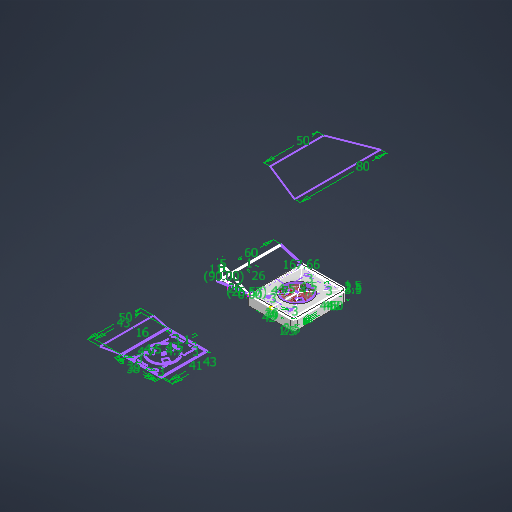
# Autodesk Inventor part: Part1
Saved by Autodesk Inventor 2026 (Build 300175000, 175)
## iProperties
Created: 2025-04-13
Part Number: Part1
Material: Generic
Document SubType Name: Modeling
Designer: ct_vi
Density: 1 g/cm^3
Appearance: Default
Author: ct_vi
Autodesk Inventor part; units mm, degrees
ref_plane "YZ Plane" through (0, 0, 0) normal (1, 0, 0) x (0, 1, 0)
ref_plane "XZ Plane" through (0, 0, 0) normal (0, 1, 0) x (-1, 0, 0)
ref_plane "XY Plane" through (0, 0, 0) normal (0, 0, 1) x (1, 0, 0)
sketch "Sketch1" plane through (0, 0, 0) normal (0, 1, 0) x (-1, 0, 0)
  circle A0 centre (0, 1.5) radius 11.5
  circle A1 centre (0, 1.5) radius 12.5
  line L0 (19.0144, -21.3297) -> (-18.8688, -21.3297) construction
  line L1 (-18.8688, -21.3297) -> (-18.8688, 21.6448) construction
  line L2 (-18.8688, 21.6448) -> (19.0144, 21.6448) construction
  line L3 (19.0144, 21.6448) -> (19.0144, -21.3297) construction
  line L4 (-2.25, -4) -> (-2.25, -8.7)
  line L5 (-2.25, -8.7) -> (2.25, -8.7)
  line L6 (2.25, -8.7) -> (2.25, -4)
  line L7 (2.25, -4) -> (-2.25, -4)
  line L8 (5.9381, 2.2148) -> (9.8353, 4.4648)
  line L9 (9.8353, 4.4648) -> (7.4853, 8.5352)
  line L10 (7.4853, 8.5352) -> (3.5881, 6.2852)
  line L11 (5.9381, 2.2148) -> (3.5881, 6.2852)
  line L12 (-3.5881, 6.2852) -> (-7.4853, 8.5352)
  line L13 (-7.4853, 8.5352) -> (-9.8353, 4.4648)
  line L14 (-9.8353, 4.4648) -> (-5.9381, 2.2148)
  line L15 (-3.5881, 6.2852) -> (-5.9381, 2.2148)
  circle A2 centre (10.199, -17.6855) radius 1.5
  circle A3 centre (-10.301, 18.0645) radius 1.5
  circle A4 centre (10.199, 18.0645) radius 1.5
  circle A5 centre (-10.301, -17.6855) radius 1.5
  line L16 (114.7256, -138.5925) -> (76.7812, -153.4955)
  line L17 (76.7812, -153.4955) -> (76.858, -73.4955)
  line L18 (76.858, -73.4955) -> (114.7256, -88.5925)
  line L19 (114.7256, -88.5925) -> (114.7256, -138.5925)
  line L20 (10.199, -17.6855) -> (-10.301, -17.6855)
  line L21 (-10.301, -17.6855) -> (-10.301, 18.0645)
  line L22 (-10.301, 18.0645) -> (10.199, 18.0645)
  line L23 (10.199, 18.0645) -> (10.199, -17.6855)
  line L24 (-4.3716, 90.6835) -> (31.6284, 90.6835)
  line L25 (31.6284, 90.6835) -> (31.6284, 131.6835)
  line L26 (31.6284, 131.6835) -> (-4.3716, 131.6835)
  line L27 (-4.3716, 131.6835) -> (-4.3716, 90.6835)
  line L28 (-4.3716, 112.6835) -> (-4.3716, 131.6835)
  circle A6 centre (13.4539, 112.6835) radius 11.5
  circle A7 centre (13.4539, 112.6835) radius 12.5
  line L29 (11.2039, 107.1835) -> (11.2039, 102.4835)
  line L30 (11.2039, 102.4835) -> (15.7039, 102.4835)
  line L31 (15.7039, 102.4835) -> (15.7039, 107.1835)
  line L32 (15.7039, 107.1835) -> (11.2039, 107.1835)
  line L33 (19.3921, 113.3983) -> (23.2892, 115.6483)
  line L34 (23.2892, 115.6483) -> (20.9392, 119.7187)
  line L35 (20.9392, 119.7187) -> (17.0421, 117.4687)
  line L36 (19.3921, 113.3983) -> (17.0421, 117.4687)
  line L37 (9.8658, 117.4687) -> (5.9687, 119.7187)
  line L38 (5.9687, 119.7187) -> (3.6187, 115.6483)
  line L39 (3.6187, 115.6483) -> (7.5158, 113.3983)
  line L40 (9.8658, 117.4687) -> (7.5158, 113.3983)
  circle A8 centre (23.6529, 93.498) radius 1.5
  circle A9 centre (3.1529, 129.248) radius 1.5
  circle A10 centre (23.6529, 129.248) radius 1.5
  circle A11 centre (3.1529, 93.498) radius 1.5
  line L41 (32.6284, 89.6835) -> (-5.3716, 89.6835)
  line L42 (-5.3716, 89.6835) -> (-5.3716, 132.6835)
  line L43 (-5.3716, 132.6835) -> (32.6284, 132.6835)
  line L44 (32.6284, 132.6835) -> (32.6284, 89.6835)
  line L45 (32.6284, 89.6835) -> (48.6284, 86.1835)
  line L46 (48.6284, 86.1835) -> (48.6284, 136.1835)
  line L47 (48.6284, 136.1835) -> (32.6284, 132.6835)
  line L48 (23.6529, 93.498) -> (3.1529, 93.498)
  line L49 (3.1529, 93.498) -> (3.1529, 129.248)
  line L50 (3.1529, 129.248) -> (23.6529, 129.248)
  line L51 (23.6529, 129.248) -> (23.6529, 93.498)
  line L52 (18, -22) -> (-18, -22)
  line L53 (-18, -22) -> (-18, 22)
  line L54 (-18, 22) -> (18, 22)
  line L55 (18, 22) -> (18, -22)
  line L56 (18, -22) -> (-18, 22) construction
  line L57 (-18, -22) -> (18, 22) construction
  line L58 (0, 0) -> (20.5, 0)
  line L59 (0, 0) -> (0, 25)
  line L60 (21, -25) -> (-17.5, -25)
  line L61 (-21, -21.5) -> (-21, 21.5)
  line L62 (-17.5, 25) -> (21, 25)
  line L63 (21, -25) -> (-21, 25) construction
  line L64 (-21, -25) -> (21, 25) construction
  arc A12 (-17.5, 25) -> (-21, 21.5) centre (-17.5, 21.5) ccw
  arc A13 (-21, -21.5) -> (-17.5, -25) centre (-17.5, -21.5) ccw
  line L65 (19, -23) -> (-17.5, -23)
  line L66 (-19, -21.5) -> (-19, 21.5)
  line L67 (-17.5, 23) -> (19, 23)
  line L68 (19, 23) -> (19, -23)
  line L69 (19, -23) -> (-19, 23) construction
  line L70 (-19, -23) -> (19, 23) construction
  arc A14 (-17.5, 23) -> (-19, 21.5) centre (-17.5, 21.5) ccw
  arc A15 (-19, -21.5) -> (-17.5, -23) centre (-17.5, -21.5) ccw
  line L71 (9.2678, 19.2405) -> (9.2678, 16.8886)
  line L72 (9.2678, -16.5095) -> (9.2678, -18.8614)
  line L73 (-9.3698, 19.2405) -> (-9.3698, 16.8886)
  line L74 (-9.3698, -16.5095) -> (-9.3698, -18.8614)
  line L75 (20, -24) -> (-17.5, -24)
  line L76 (-20, -21.5) -> (-20, 21.5)
  line L77 (-17.5, 24) -> (20, 24)
  line L78 (20, -24) -> (-20, 24) construction
  line L79 (-20, -24) -> (20, 24) construction
  arc A16 (-17.5, 24) -> (-20, 21.5) centre (-17.5, 21.5) ccw
  arc A17 (-20, -21.5) -> (-17.5, -24) centre (-17.5, -21.5) ccw
  line L80 (21, -25) -> (47, -30.85)
  line L81 (47, -30.85) -> (47, 29.15)
  line L82 (47, 29.15) -> (21, 25)
  line L83 (24.0357, 24.4719) -> (46, 27.9777)
  line L84 (46, 27.9777) -> (46, -29.6)
  line L85 (46, -29.6) -> (21.2195, -24.0244)
  line L86 (20, 24) -> (21, 24)
  line L87 (21, 24) -> (21.1111, 24)
  line L88 (21, 24) -> (21.1111, 24) construction
  line L89 (24.0357, 24.4719) -> (21.1111, 24)
  line L90 (21.2195, -24.0244) -> (21.2854, -24.0244) construction
  line L91 (21.2195, -24.0244) -> (21.108, -24)
  line L92 (21.2195, -24.0244) -> (21.3336, -24.0244) construction
  line L93 (21.108, -24) -> (20, -24)
  line L94 (21, -25) -> (21, 25)
  line L95 (19, -23) -> (21, -23)
  line L96 (19, 23) -> (21, 23)
  line L97 (19, 24) -> (19, 23)
  line L98 (19, -23) -> (19, -24)
  point P0 (13.4539, 111.1835)
  point P1 (21, -22)
  point P2 (21, 22)
  point P3 (21, -24)
  dimension "d33" = 4.7
  dimension "d34" = 4.5
  dimension "d36" = 4.5
  dimension "d37" = 4.7
  dimension "d38" = 3
  dimension "d46" = 3
  dimension "d47" = 3
  dimension "d48" = 3
  dimension "d88" = 80
  dimension "d89" = 50
  dimension "d136" = 4.7
  dimension "d137" = 4.5
  dimension "d138" = 4.5
  dimension "d139" = 4.7
  dimension "d140" = 3
  dimension "d141" = 3
  dimension "d142" = 3
  dimension "d143" = 3
  dimension "d144" = 1
  dimension "d145" = 41
  dimension "d146" = 43
  dimension "d147" = 43
  dimension "d148" = 50
  dimension "d149" = 38
  dimension "d150" = 36
  dimension "d151" = 16
  dimension "d159" = 36
  dimension "d165" = 42
  dimension "d166" = 50
  dimension "d170" = 38
  dimension "d192" = 40
  dimension "d193" = 48
  dimension "d209" = 60
  dimension "d210" = 46
  dimension "d211" = 1.5
  dimension "d212" = 2.5
  dimension "d213" = 1.5
  dimension "d214" = 2.5
  dimension "d215" = 3.5
  dimension "d216" = 3.5
  dimension "d217" = 44
  dimension "d219" = 1
  dimension "d220" = 0
  dimension "d222" = 167.66
  dimension "d236" = 26
  constraints: 190 end point, 27 perpendicular, 23 point on line, 20 point on circle, 18 centre point, 12 horizontal, 12 parallel, 12 tangent, 8 midpoint, 4 equal length, 3 vertical, 4 other
  measures "d33" distance of L4.start L4.end
  measures "d34" distance of L4.end L5.end
  measures "d36" distance of L8.start L8.end
  measures "d37" distance of L8.end L9.end
  measures "d38" diameter of A2
  measures "d46" diameter of A3
  measures "d47" diameter of A4
  measures "d48" diameter of A5
  measures "d88" distance of L16.end L17.end
  measures "d89" distance of L18.end L16.start
  measures "d136" distance of L29.start L29.end
  measures "d137" distance of L29.end L30.end
  measures "d138" distance of L33.start L33.end
  measures "d139" distance of L33.end L34.end
  measures "d140" diameter of A8
  measures "d141" diameter of A9
  measures "d142" diameter of A10
  measures "d143" diameter of A11
  measures "d144" distance between parallel lines of L24 L41
  measures "d145" distance of L26.end L24.start
  measures "d146" distance of L42.start L43.start
  measures "d147" distance of L43.end L44.end
  measures "d148" distance of L45.end L47.start
  measures "d149" distance of L43.start L43.end
  measures "d150" distance of L26.start L26.end
  measures "d151" distance between parallel lines of L44 L46
  measures "d159" distance of L53.end L54.end
  measures "d165" distance of L63.end L62.end
  measures "d166" distance of L64.start L63.end
  measures "d170" distance of L69.end L67.end
  measures "d192" distance of L78.end L77.end
  measures "d193" distance of L79.start L78.end
  measures "d209" distance of L80.end L81.end
  measures "d210" distance between parallel lines of L67 L65
  measures "d211" radius of A15
  measures "d212" radius of A17
  measures "d213" radius of A14
  measures "d214" radius of A16
  measures "d215" radius of A12
  measures "d216" radius of A13
  measures "d217" distance between parallel lines of L54 L52
  measures "d219" distance between parallel lines of L81 L84
  measures "d220" distance between parallel lines of L88 L87
  measures "d222" angle of L92 L91
  measures "d236" distance between parallel lines of L94 L81
extrude "Extrusion1" add sketch "Sketch1" against normal blind 2.5 contours A0 L23 A1 L58 | A0 L59 A1 L23 | L58 A1 L23 A0 | A0 L21 A1 L59 | L23 A1 L21 A0 | A0 L21 A1
extrude "Extrusion4" add sketch "Sketch1" against normal blind 5 contours L23 L22 L71 A4 | A4 L71 L22 L23 | A4 L22 L71 | L23 L20 L72 A2 | A2 L72 L20 L23 | L21 L22 L73 A3 | A3 L73 L22 L21 | L22 L73 A3 | A3 L73 L22 | A4 L71 L22 | L21 L20 L74 A5 | A5 L74 L20 L21 | L72 L20 A2 | A5 L20 L74 | L74 L20 A5 | A2 L20 L72
extrude "Extrusion11" add sketch "Sketch1" against normal blind 1 contours L23 A4 L22 L59 L54 L55 L58 A1 | A1 L59 L22 A4 L23 | L58 L55 L52 L53 L54 L59 L22 A3 L21 A1 A5 L20 A2 L23 | A1 L21 A3 L22 L59 | L23 A2 L20 A5 L21 A1
extrude "Extrusion13" add sketch "Sketch1" along normal blind 0.5 contours A0 L23 A1 L58 | A0 L59 A1 L23 | L58 A1 L23 A0 | A0 L21 A1 L59 | L23 A4 L22 L59 L54 L55 L58 A1 | A1 L59 L22 A4 L23 | L23 A1 L21 A0 | L58 L55 L52 L53 L54 L59 L22 A3 L21 A1 A5 L20 A2 L23 | A0 L21 A1 | A1 L21 A3 L22 L59 | L23 L22 L71 A4 | A4 L71 L22 L23 | L23 A2 L20 A5 L21 A1 | L58 L68 L65 A15 L66 A14 L67 L59 L54 L53 L52 L55 | L55 L54 L59 L67 L68 L58 | A4 L22 L71 | L23 L20 L72 A2 | A2 L72 L20 L23 | L21 L22 L73 A3 | A3 L73 L22 L21 | L22 L73 A3 | A3 L73 L22 | A4 L71 L22 | L21 L20 L74 A5 | A5 L74 L20 L21 | L72 L20 A2 | A5 L20 L74 | L74 L20 A5 | A2 L20 L72
extrude "Extrusion15" add sketch "Sketch1" against normal blind 1 contours L58 L68 L65 A15 L66 A14 L67 L59 L54 L53 L52 L55 | L55 L54 L59 L67 L68 L58
extrude "Extrusion16" cut sketch "Sketch1" against normal through all contours A4 L22 L71 | L22 L73 A3 | A3 L73 L22 | A4 L71 L22 | L72 L20 A2 | A5 L20 L74 | L74 L20 A5 | A2 L20 L72
extrude "Extrusion17" [suppressed]
extrude "Extrusion14" [suppressed]
fillet "Fillet5" [suppressed]
chamfer "Chamfer1" distance 1.5 angle 45 1 edges at (11.5, 0.5, 1.5)
extrude "Extrusion18" add sketch "Sketch1" along normal blind 0.5 and the other way blind 7 contours L67 L59 L77 L97 | L98 L75 A17 L76 A16 L77 L59 L67 A14 L66 A15 L65
extrude "Extrusion19" add sketch "Sketch1" along normal blind 0.5 and the other way blind 1 contours L68 L96 L94 L95 | L97 L77 L86 L94 L96 | L95 L94 L93 L75 L98
extrude "Extrusion20" [suppressed]
extrude "Extrusion21" add sketch "Sketch1" against normal blind 9 contours L77 L59 L62 L94 L86 | L75 L93 L94 L60 A13 L61 A12 L62 L59 L77 A16 L76 A17
sketch "Sketch3" plane through (-21, 0, 25) normal (0, 0, 1) x (1, 0, 0)
  line L0 (0, 0) -> (0, 0.5) projected
  line L1 (0, 0) -> (0, 0.5)
  line L2 (0, 0) -> (-26, 0)
  line L3 (-26, 0) -> (-26, 11)
  line L4 (-26, 0) -> (-15, 0) construction
  line L5 (-26, 11) -> (-21, 11)
  line L6 (-21, 11) -> (0, 0.5)
  line L7 (0, 0.5) -> (0.4617, 0.5)
  line L8 (-21.2361, 10) -> (-25, 10)
  line L9 (-25, 10) -> (-25, 1)
  line L10 (-25, 1) -> (-3.2361, 1)
  line L11 (-3.2361, 1) -> (-21.2361, 10)
  point P0 (21, 0)
  point P1 (-20, 0)
  dimension "d237" = 26
  dimension "d238" = 11
  dimension "d239" = 90
  dimension "d240" = 5
  dimension "d241" = 26.565
  dimension "d242" = 1
  constraints: 22 end point, 3 horizontal, 3 perpendicular, 2 vertical, 3 other
  measures "d237" distance of L0.start L2.end
  measures "d238" distance of L2.end L3.end
  measures "d239" angle of L4 L3
  measures "d240" distance of L3.end L5.end
  measures "d241" angle of L7 L6
  measures "d242" distance between parallel lines of L5 L8
body "Solid1"
